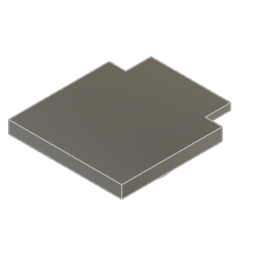
Case (Autodesk Fusion 360 archive; units mm, degrees)
design "Etiquette_game"
Autodesk Fusion 360 part; units mm, degrees
(part 1 of 2)
sketch "Esquisse1" plane through (0, 0, 0) normal (0, 1, 0) x (1, 0, 0)
  line L0 (0, 0) -> (9.5, 0)
  line L1 (9.5, 0) -> (9.5, 0.8)
  line L2 (9.5, 0.8) -> (0, 0.8)
  line L3 (0, 0.8) -> (0, 0)
  dimension "d1" = 9.5
  dimension "d2" = 0.8
  constraint horizontal L0
  constraint vertical L1
  constraint horizontal L2
  constraint vertical L3
  constraint coincident L0.start L3.end
  measures "d1" distance of L0.start L0.end
  measures "d2" distance of L0.start L2.end
extrude "Extrusion1" add sketch "Esquisse1" along normal blind 3
sketch "Esquisse2" plane through (0, 0, 0) normal (0, -1, 0) x (1, 0, 0)
  line L0 (0, 0) -> (0, -0.8)
  line L1 (0, -0.8) -> (9.5, -0.8)
  line L2 (9.5, -0.8) -> (9.5, 0)
  line L3 (9.5, 0) -> (0, 0)
  line L4 (0, 0) -> (-2, 0) construction
  line L5 (9.5, 0) -> (11.5, 0)
  line L6 (11.5, 0) -> (11.5, -1.5)
  line L7 (-2, 0) -> (11.5, 0)
  line L8 (11.5, 0) -> (11.5, -1.5)
  line L9 (11.5, -1.5) -> (-2, -1.5)
  line L10 (-2, -1.5) -> (-2, 0)
  dimension "d5" = 2
  dimension "d6" = 2
  dimension "d7" = 1.5
  constraint coincident L0.start L3.end
  constraint perpendicular L0 L4
  constraint coincident L2.end L3.start
  constraint perpendicular L2 L5
  constraint perpendicular L5 L6
  constraint horizontal L7
  constraint vertical L8
  constraint horizontal L9
  constraint vertical L10
  measures "d5" distance of L0.start L4.end
  measures "d6" distance of L2.end L5.end
  measures "d7" distance of L5.end L6.end
extrude "Extrusion2" add sketch "Esquisse2" along normal blind 12
sketch "Esquisse3" plane through (0, 0, -1.5) normal (0, 0, -1) x (1, 0, 0)
  line L0 (-2, 0) -> (11.5, 0)
  line L1 (11.5, 0) -> (11.5, 12)
  line L2 (11.5, 12) -> (-2, 12)
  line L3 (-2, 12) -> (-2, 0)
  line L4 (0, 6.6162) -> (4, 6.6162)
  line L5 (4, 6.6162) -> (4, 5.4162)
  line L6 (4, 5.4162) -> (0, 5.4162)
  line L7 (0, 5.4162) -> (0, 6.6162)
  line L8 (0, 5.4162) -> (1.4, 5.4162)
  line L9 (1.4, 5.4162) -> (2.6, 5.4162)
  line L10 (2.6, 5.4162) -> (2.6, 4.0162)
  line L11 (2.6, 4.0162) -> (1.4, 4.0162)
  line L12 (1.4, 4.0162) -> (1.4, 5.4162)
  line L13 (1.4, 4.0162) -> (2.6, 4.0162)
  line L14 (2.6, 4.0162) -> (2.6, 8.0162)
  line L15 (2.6, 8.0162) -> (1.4, 8.0162)
  line L16 (1.4, 8.0162) -> (1.4, 4.0162)
  circle A0 centre (6.7088, 5.2403) radius 0.85
  circle A1 centre (8.2624, 6.7784) radius 0.85
  arc A2 (1.5165, 9.1275) -> (4.0468, 3.6361) centre (2.0261, 6.0336) ccw
  line L17 (1.5165, 9.1275) -> (7.8999, 9.1275)
  line L18 (4.0468, 3.6361) -> (5.4235, 3.6361)
  arc A3 (5.4235, 3.6361) -> (7.8999, 9.1275) centre (7.4769, 6.0141) ccw
  dimension "d10" = 4
  dimension "d11" = 1.2
  dimension "d12" = 1.4
  dimension "d13" = 1.2
  dimension "d14" = 1.4
  dimension "d15" = 1.2
  dimension "d16" = 4
  dimension "d17" = 1.7
  dimension "d18" = 1.7
  constraint horizontal L4
  constraint vertical L5
  constraint horizontal L6
  constraint vertical L7
  constraint perpendicular L7 L8
  constraint horizontal L9
  constraint vertical L10
  constraint horizontal L11
  constraint vertical L12
  constraint horizontal L13
  constraint vertical L14
  constraint horizontal L15
  constraint vertical L16
  constraint horizontal L17
  constraint horizontal L18
  measures "d10" distance of L4.start L4.end
  measures "d11" distance of L4.start L6.end
  measures "d12" distance of L6.end L8.end
  measures "d13" distance of L8.end L9.end
  measures "d14" distance of L8.end L11.end
  measures "d15" distance of L11.end L10.end
  measures "d16" distance of L11.end L15.end
  measures "d17" diameter of A0
  measures "d18" diameter of A1
extrude "Extrusion3" add sketch "Esquisse3" along normal blind 1 contours A2 L17 L18 A3

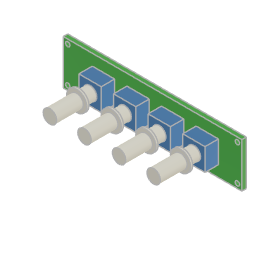
design "PCB_potar"
Autodesk Fusion 360 part; units mm, degrees
sketch "Esquisse1" plane through (0, 0, 0) normal (0, 1, 0) x (1, 0, 0)
  line L0 (0, 0) -> (80, 0)
  line L1 (80, 0) -> (80, 20)
  line L2 (80, 20) -> (0, 20)
  line L3 (0, 20) -> (0, 0)
  line L4 (0, 20) -> (2, 20) construction
  line L5 (2, 20) -> (2, 18) construction
  line L6 (2, 18) -> (0, 18) construction
  line L7 (0, 18) -> (0, 20) construction
  line L8 (0, 0) -> (2, 0) construction
  line L9 (2, 0) -> (2, 2) construction
  line L10 (2, 2) -> (0, 2) construction
  line L11 (0, 2) -> (0, 0) construction
  circle A0 centre (2, 2) radius 1
  circle A1 centre (2, 18) radius 1
  line L12 (40, 20) -> (40, 0) construction
  circle A2 centre (78, 2) radius 1
  circle A3 centre (78, 18) radius 1
  dimension "d1" = 80
  dimension "d2" = 20
  dimension "d20" = 2
  dimension "d21" = 2
  dimension "d22" = 2
  dimension "d23" = 2
  dimension "d24" = 2
  dimension "d25" = 2
  constraint horizontal L0
  constraint vertical L1
  constraint horizontal L2
  constraint vertical L3
  constraint coincident L0.start L3.end
  constraint horizontal L4
  constraint vertical L5
  constraint horizontal L6
  constraint vertical L7
  constraint horizontal L8
  constraint vertical L9
  constraint horizontal L10
  constraint vertical L11
  constraint coincident L9.end L10.start
  constraint coincident L5.end L6.start
  constraint midpoint L2 L12.start
  constraint midpoint L0 L12.end
  constraint symmetric A0 L12 A2
  constraint symmetric A1 L12 A3
  measures "d1" distance of L0.start L0.end
  measures "d2" distance of L0.start L2.end
  measures "d20" distance of L2.end L4.end
  measures "d21" distance of L2.end L6.end
  measures "d22" distance of L0.start L8.end
  measures "d23" distance of L0.start L10.end
  measures "d24" diameter of A0
  measures "d25" diameter of A1
extrude "Extrusion1" add sketch "Esquisse1" along normal blind 2 makes body 1
sketch "Esquisse2" plane through (0, 0, 0) normal (0, -1, 0) x (1, 0, 0)
  line L0 (0, 0) -> (0, -20)
  line L1 (0, -20) -> (80, -20)
  line L2 (80, -20) -> (80, 0)
  line L3 (80, 0) -> (0, 0)
  line L4 (0, 0) -> (13, 0) construction
  line L5 (13, 0) -> (13, -5) construction
  line L6 (13, -5) -> (23, -5)
  line L7 (23, -5) -> (23, -15)
  line L8 (23, -15) -> (13, -15)
  line L9 (13, -15) -> (13, -5)
  line L10 (23, -5) -> (28.5, -5) construction
  line L11 (28.5, -5) -> (38.5, -5)
  line L12 (38.5, -5) -> (38.5, -15)
  line L13 (38.5, -15) -> (28.5, -15)
  line L14 (28.5, -15) -> (28.5, -5)
  line L15 (38.5, -5) -> (44, -5) construction
  line L16 (44, -5) -> (54, -5)
  line L17 (54, -5) -> (54, -15)
  line L18 (54, -15) -> (44, -15)
  line L19 (44, -15) -> (44, -5)
  line L20 (54, -5) -> (59.5, -5) construction
  line L21 (59.5, -5) -> (69.5, -5)
  line L22 (69.5, -5) -> (69.5, -15)
  line L23 (69.5, -15) -> (59.5, -15)
  line L24 (59.5, -15) -> (59.5, -5)
  circle A0 centre (78, -2) radius 1
  circle A1 centre (2, -18) radius 1
  circle A2 centre (2, -2) radius 1
  circle A3 centre (78, -18) radius 1
  dimension "d5" = 13
  dimension "d6" = 5
  dimension "d7" = 10
  dimension "d8" = 10
  dimension "d9" = 5.5
  dimension "d10" = 10
  dimension "d11" = 10
  dimension "d12" = 5.5
  dimension "d13" = 10
  dimension "d14" = 10
  dimension "d15" = 5.5
  dimension "d16" = 10
  dimension "d17" = 10
  constraint coincident L0.start L3.end
  constraint perpendicular L0 L4
  constraint perpendicular L1 L5
  constraint horizontal L6
  constraint vertical L7
  constraint horizontal L8
  constraint vertical L9
  constraint perpendicular L7 L10
  constraint horizontal L11
  constraint vertical L12
  constraint horizontal L13
  constraint vertical L14
  constraint perpendicular L12 L15
  constraint horizontal L16
  constraint vertical L17
  constraint horizontal L18
  constraint vertical L19
  constraint perpendicular L17 L20
  constraint horizontal L21
  constraint vertical L22
  constraint horizontal L23
  constraint vertical L24
  measures "d5" distance of L0.start L4.end
  measures "d6" distance of L4.end L5.end
  measures "d7" distance of L5.end L6.end
  measures "d8" distance of L5.end L8.end
  measures "d9" distance of L6.end L10.end
  measures "d10" distance of L10.end L11.end
  measures "d11" distance of L10.end L13.end
  measures "d12" distance of L11.end L15.end
  measures "d13" distance of L15.end L16.end
  measures "d14" distance of L15.end L18.end
  measures "d15" distance of L16.end L20.end
  measures "d16" distance of L20.end L21.end
  measures "d17" distance of L20.end L23.end
extrude "Extrusion2" add sketch "Esquisse2" along normal blind 6 separate body contours L6 L7 L8 L9 | L11 L12 L13 L14 | L16 L17 L18 L19 | L21 L22 L23 L24 makes body 2 at (31.8333, 0, -8.3333) makes body 3 at (47.3333, 0, -11.6667) makes body 4 at (16.3333, 0, -8.3333) makes body 5 at (62.8333, 0, -8.3333)
sketch "Esquisse3" plane through (0, -6, 0) normal (0, -1, 0) x (1, 0, 0)
  line L0 (13, -15) -> (23, -15)
  line L1 (23, -15) -> (23, -5)
  line L2 (23, -5) -> (13, -5)
  line L3 (13, -5) -> (13, -15)
  line L4 (13, -5) -> (23, -15) construction
  line L5 (13, -15) -> (23, -5) construction
  circle A0 centre (18, -10) radius 3
  dimension "d26" = 6
  constraint coincident L2.end L3.start
  constraint coincident L0.end L1.start
  constraint coincident L0.start L3.end
  constraint coincident L1.end L2.start
  constraint midpoint L5 A0.centre
  measures "d26" diameter of A0
extrude "Extrusion3" add sketch "Esquisse3" along normal blind 5 separate body contours A0 makes body 6
sketch "Esquisse4" plane through (0, -11, 0) normal (0, -1, 0) x (1, 0, 0)
  circle A0 centre (18, -10) radius 3
  circle A1 centre (18, -10) radius 4.5
  dimension "d29" = 9
  constraint concentric A0 A1
  measures "d29" diameter of A1
extrude "Extrusion4" add sketch "Esquisse4" along normal blind 1 contours A0 | A1 bodies 6
sketch "Esquisse5" plane through (0, -12, 0) normal (0, -1, 0) x (1, 0, 0)
  circle A0 centre (18, -10) radius 4.5
  circle A1 centre (18, -10) radius 3
  dimension "d32" = 6
  constraint concentric A0 A1
  measures "d32" diameter of A1
extrude "Extrusion5" add sketch "Esquisse5" along normal blind 12 contours A1 bodies 6
copy_body "Copier/Coller des corps1" bodies 6 makes body 7
move_body "Déplacer1" bodies 7 to x (1, 0, 0) y (0, 1, 0) z (0, 0, 1) at (15.5, 0, 0)
copy_body "Copier/Coller des corps2" bodies 6 makes body 8
move_body "Déplacer2" bodies 8 to x (1, 0, 0) y (0, 1, 0) z (0, 0, 1) at (31, 0, 0)
copy_body "Copier/Coller des corps3" bodies 6 makes body 9
move_body "Déplacer3" bodies 9 to x (1, 0, 0) y (0, 1, 0) z (0, 0, 1) at (46.5, 0, 0)
named bodies: "BASE_PCB", "POTAR_1", "POTAR_2", "POTAR_3", "POTAR_4", "KNOB_1", "KNOB_2", "KNOB_1 (1)", "KNOB_3", "KNOB_1 (2)", "KNOB_4"

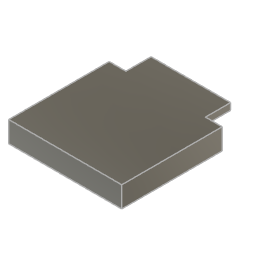
design "Etiquette_deezer"
Autodesk Fusion 360 part; units mm, degrees
sketch "Esquisse1" plane through (0, 0, 0) normal (0, 1, 0) x (1, 0, 0)
  line L0 (0, 0) -> (9.5, 0)
  line L1 (9.5, 0) -> (9.5, 0.8)
  line L2 (9.5, 0.8) -> (0, 0.8)
  line L3 (0, 0.8) -> (0, 0)
  dimension "d1" = 9.5
  dimension "d2" = 0.8
  constraint horizontal L0
  constraint vertical L1
  constraint horizontal L2
  constraint vertical L3
  constraint coincident L0.start L3.end
  measures "d1" distance of L0.start L0.end
  measures "d2" distance of L0.start L2.end
extrude "Extrusion1" add sketch "Esquisse1" along normal blind 3
sketch "Esquisse2" plane through (0, 0, 0) normal (0, -1, 0) x (1, 0, 0)
  line L0 (0, 0) -> (0, -0.8)
  line L1 (0, -0.8) -> (9.5, -0.8)
  line L2 (9.5, -0.8) -> (9.5, 0)
  line L3 (9.5, 0) -> (0, 0)
  line L4 (0, 0) -> (-2, 0) construction
  line L5 (9.5, 0) -> (11.5, 0)
  line L6 (11.5, 0) -> (11.5, -1.5)
  line L7 (-2, 0) -> (11.5, 0)
  line L8 (11.5, 0) -> (11.5, -1.5)
  line L9 (11.5, -1.5) -> (-2, -1.5)
  line L10 (-2, -1.5) -> (-2, 0)
  dimension "d5" = 2
  dimension "d6" = 2
  dimension "d7" = 1.5
  constraint coincident L0.start L3.end
  constraint perpendicular L0 L4
  constraint coincident L2.end L3.start
  constraint perpendicular L2 L5
  constraint perpendicular L5 L6
  constraint horizontal L7
  constraint vertical L8
  constraint horizontal L9
  constraint vertical L10
  measures "d5" distance of L0.start L4.end
  measures "d6" distance of L2.end L5.end
  measures "d7" distance of L5.end L6.end
extrude "Extrusion2" add sketch "Esquisse2" along normal blind 12
sketch "Esquisse3" plane through (0, 0, -1.5) normal (0, 0, -1) x (1, 0, 0)
  line L0 (-2, 0) -> (11.5, 0)
  line L1 (11.5, 0) -> (11.5, 12)
  line L2 (11.5, 12) -> (-2, 12)
  line L3 (-2, 12) -> (-2, 0)
  line L4 (-2, 12) -> (11.5, 0) construction
  line L5 (-2, 0) -> (11.5, 12) construction
  circle A0 centre (4.75, 6) radius 5.5
  line L6 (0.5787, 3.684) -> (2.1287, 3.684)
  line L7 (2.1287, 3.684) -> (2.1287, 4.184)
  line L8 (2.1287, 4.184) -> (0.5787, 4.184)
  line L9 (0.5787, 4.184) -> (0.5787, 3.684)
  line L10 (0.5787, 4.184) -> (0.5787, 4.254)
  line L11 (0.5787, 4.254) -> (2.1287, 4.254)
  line L12 (2.1287, 4.254) -> (2.1287, 4.754)
  line L13 (2.1287, 4.754) -> (0.5787, 4.754)
  line L14 (0.5787, 4.754) -> (0.5787, 4.254)
  line L15 (0.5787, 4.754) -> (0.5787, 4.824)
  line L16 (0.5787, 4.824) -> (2.1287, 4.824)
  line L17 (2.1287, 4.824) -> (2.1287, 5.324)
  line L18 (2.1287, 5.324) -> (0.5787, 5.324)
  line L19 (0.5787, 5.324) -> (0.5787, 4.824)
  line L20 (0.5787, 5.324) -> (0.5787, 5.394)
  line L21 (0.5787, 5.394) -> (2.1287, 5.394)
  line L22 (2.1287, 5.394) -> (2.1287, 5.894)
  line L23 (2.1287, 5.894) -> (0.5787, 5.894)
  line L24 (0.5787, 5.894) -> (0.5787, 5.394)
  line L25 (0.5787, 5.894) -> (0.5787, 5.964)
  line L26 (0.5787, 5.964) -> (2.1287, 5.964)
  line L27 (2.1287, 5.964) -> (2.1287, 6.464)
  line L28 (2.1287, 6.464) -> (0.5787, 6.464)
  line L29 (0.5787, 6.464) -> (0.5787, 5.964)
  line L30 (8.9164, 5.394) -> (8.9164, 5.894)
  line L31 (8.9164, 4.824) -> (8.9164, 5.324)
  line L32 (7.3664, 4.184) -> (7.3664, 3.684)
  line L33 (8.9164, 3.684) -> (8.9164, 4.184)
  line L34 (8.9164, 5.324) -> (7.3664, 5.324)
  line L35 (8.9164, 4.754) -> (7.3664, 4.754)
  line L36 (8.9164, 4.254) -> (8.9164, 4.754)
  line L37 (7.3664, 6.464) -> (7.3664, 5.964)
  line L38 (7.3664, 4.754) -> (7.3664, 4.254)
  line L39 (7.3664, 5.894) -> (7.3664, 5.394)
  line L40 (8.9164, 5.964) -> (8.9164, 6.464)
  line L41 (7.3664, 4.754) -> (7.3664, 4.824)
  line L42 (7.3664, 5.324) -> (7.3664, 5.394)
  line L43 (7.3664, 5.324) -> (7.3664, 4.824)
  line L44 (8.9164, 5.894) -> (7.3664, 5.894)
  line L45 (7.3664, 3.684) -> (8.9164, 3.684)
  line L46 (7.3664, 4.254) -> (8.9164, 4.254)
  line L47 (7.3664, 5.394) -> (8.9164, 5.394)
  line L48 (7.3664, 4.824) -> (8.9164, 4.824)
  line L49 (7.3664, 4.184) -> (7.3664, 4.254)
  line L50 (8.9164, 4.184) -> (7.3664, 4.184)
  line L51 (8.9164, 6.464) -> (7.3664, 6.464)
  line L52 (7.3664, 5.894) -> (7.3664, 5.964)
  line L53 (7.3664, 5.964) -> (8.9164, 5.964)
  line L54 (5.5066, 5.394) -> (5.5066, 5.894)
  line L55 (5.5066, 4.824) -> (5.5066, 5.324)
  line L56 (3.9566, 4.184) -> (3.9566, 3.684)
  line L57 (5.5066, 3.684) -> (5.5066, 4.184)
  line L58 (5.5066, 5.324) -> (3.9566, 5.324)
  line L59 (5.5066, 4.754) -> (3.9566, 4.754)
  line L60 (5.5066, 4.254) -> (5.5066, 4.754)
  line L61 (3.9566, 6.464) -> (3.9566, 5.964)
  line L62 (3.9566, 4.754) -> (3.9566, 4.254)
  line L63 (3.9566, 5.894) -> (3.9566, 5.394)
  line L64 (5.5066, 5.964) -> (5.5066, 6.464)
  line L65 (3.9566, 4.754) -> (3.9566, 4.824)
  line L66 (3.9566, 5.324) -> (3.9566, 5.394)
  line L67 (3.9566, 5.324) -> (3.9566, 4.824)
  line L68 (5.5066, 5.894) -> (3.9566, 5.894)
  line L69 (3.9566, 3.684) -> (5.5066, 3.684)
  line L70 (3.9566, 4.254) -> (5.5066, 4.254)
  line L71 (3.9566, 5.394) -> (5.5066, 5.394)
  line L72 (3.9566, 4.824) -> (5.5066, 4.824)
  line L73 (3.9566, 4.184) -> (3.9566, 4.254)
  line L74 (5.5066, 4.184) -> (3.9566, 4.184)
  line L75 (5.5066, 6.464) -> (3.9566, 6.464)
  line L76 (3.9566, 5.894) -> (3.9566, 5.964)
  line L77 (3.9566, 5.964) -> (5.5066, 5.964)
  line L78 (7.1756, 5.394) -> (7.1756, 5.894)
  line L79 (7.1756, 4.824) -> (7.1756, 5.324)
  line L80 (5.6256, 4.184) -> (5.6256, 3.684)
  line L81 (7.1756, 3.684) -> (7.1756, 4.184)
  line L82 (7.1756, 5.324) -> (5.6256, 5.324)
  line L83 (7.1756, 4.754) -> (5.6256, 4.754)
  line L84 (7.1756, 4.254) -> (7.1756, 4.754)
  line L85 (5.6256, 6.464) -> (5.6256, 5.964)
  line L86 (5.6256, 4.754) -> (5.6256, 4.254)
  line L87 (5.6256, 5.894) -> (5.6256, 5.394)
  line L88 (7.1756, 5.964) -> (7.1756, 6.464)
  line L89 (5.6256, 4.754) -> (5.6256, 4.824)
  line L90 (5.6256, 5.324) -> (5.6256, 5.394)
  line L91 (5.6256, 5.324) -> (5.6256, 4.824)
  line L92 (7.1756, 5.894) -> (5.6256, 5.894)
  line L93 (5.6256, 3.684) -> (7.1756, 3.684)
  line L94 (5.6256, 4.254) -> (7.1756, 4.254)
  line L95 (5.6256, 5.394) -> (7.1756, 5.394)
  line L96 (5.6256, 4.824) -> (7.1756, 4.824)
  line L97 (5.6256, 4.184) -> (5.6256, 4.254)
  line L98 (7.1756, 4.184) -> (5.6256, 4.184)
  line L99 (7.1756, 6.464) -> (5.6256, 6.464)
  line L100 (5.6256, 5.894) -> (5.6256, 5.964)
  line L101 (5.6256, 5.964) -> (7.1756, 5.964)
  line L102 (3.8376, 5.394) -> (3.8376, 5.894)
  line L103 (3.8376, 4.824) -> (3.8376, 5.324)
  line L104 (2.2876, 4.184) -> (2.2876, 3.684)
  line L105 (3.8376, 3.684) -> (3.8376, 4.184)
  line L106 (3.8376, 5.324) -> (2.2876, 5.324)
  line L107 (3.8376, 4.754) -> (2.2876, 4.754)
  line L108 (3.8376, 4.254) -> (3.8376, 4.754)
  line L109 (2.2876, 6.464) -> (2.2876, 5.964)
  line L110 (2.2876, 4.754) -> (2.2876, 4.254)
  line L111 (2.2876, 5.894) -> (2.2876, 5.394)
  line L112 (3.8376, 5.964) -> (3.8376, 6.464)
  line L113 (2.2876, 4.754) -> (2.2876, 4.824)
  line L114 (2.2876, 5.324) -> (2.2876, 5.394)
  line L115 (2.2876, 5.324) -> (2.2876, 4.824)
  line L116 (3.8376, 5.894) -> (2.2876, 5.894)
  line L117 (2.2876, 3.684) -> (3.8376, 3.684)
  line L118 (2.2876, 4.254) -> (3.8376, 4.254)
  line L119 (2.2876, 5.394) -> (3.8376, 5.394)
  line L120 (2.2876, 4.824) -> (3.8376, 4.824)
  line L121 (2.2876, 4.184) -> (2.2876, 4.254)
  line L122 (3.8376, 4.184) -> (2.2876, 4.184)
  line L123 (3.8376, 6.464) -> (2.2876, 6.464)
  line L124 (2.2876, 5.894) -> (2.2876, 5.964)
  line L125 (2.2876, 5.964) -> (3.8376, 5.964)
  line L126 (5.507, 5.3964) -> (5.507, 5.8964)
  line L127 (3.957, 4.8264) -> (5.507, 4.8264)
  line L128 (5.507, 5.3264) -> (3.957, 5.3264)
  line L129 (5.507, 4.8264) -> (5.507, 5.3264)
  line L130 (3.957, 7.1064) -> (5.507, 7.1064)
  line L131 (3.957, 6.4664) -> (3.957, 6.5364)
  line L132 (5.507, 7.6064) -> (3.957, 7.6064)
  line L133 (5.507, 6.5364) -> (5.507, 7.0364)
  line L134 (3.957, 7.6064) -> (3.957, 7.1064)
  line L135 (5.507, 6.4664) -> (3.957, 6.4664)
  line L136 (5.507, 7.0364) -> (3.957, 7.0364)
  line L137 (5.507, 5.8964) -> (3.957, 5.8964)
  line L138 (3.957, 5.3964) -> (5.507, 5.3964)
  line L139 (5.507, 7.1064) -> (5.507, 7.6064)
  line L140 (3.957, 7.0364) -> (3.957, 6.5364)
  line L141 (3.957, 7.0364) -> (3.957, 7.1064)
  line L142 (3.957, 6.4664) -> (3.957, 5.9664)
  line L143 (3.957, 5.9664) -> (5.507, 5.9664)
  line L144 (3.957, 5.8964) -> (3.957, 5.9664)
  line L145 (3.957, 5.3264) -> (3.957, 5.3964)
  line L146 (5.507, 5.9664) -> (5.507, 6.4664)
  line L147 (3.957, 5.8964) -> (3.957, 5.3964)
  line L148 (3.957, 5.3264) -> (3.957, 4.8264)
  line L149 (3.957, 6.5364) -> (5.507, 6.5364)
  line L150 (8.9062, 7.2438) -> (8.9062, 7.7438)
  line L151 (7.3562, 6.6738) -> (8.9062, 6.6738)
  line L152 (8.9062, 7.1738) -> (7.3562, 7.1738)
  line L153 (8.9062, 6.6738) -> (8.9062, 7.1738)
  line L154 (7.3562, 8.9538) -> (8.9062, 8.9538)
  line L155 (7.3562, 8.3138) -> (7.3562, 8.3838)
  line L156 (8.9062, 9.4538) -> (7.3562, 9.4538)
  line L157 (8.9062, 8.3838) -> (8.9062, 8.8838)
  line L158 (7.3562, 9.4538) -> (7.3562, 8.9538)
  line L159 (8.9062, 8.3138) -> (7.3562, 8.3138)
  line L160 (8.9062, 8.8838) -> (7.3562, 8.8838)
  line L161 (8.9062, 7.7438) -> (7.3562, 7.7438)
  line L162 (7.3562, 7.2438) -> (8.9062, 7.2438)
  line L163 (8.9062, 8.9538) -> (8.9062, 9.4538)
  line L164 (7.3562, 8.8838) -> (7.3562, 8.3838)
  line L165 (7.3562, 8.8838) -> (7.3562, 8.9538)
  line L166 (7.3562, 8.3138) -> (7.3562, 7.8138)
  line L167 (7.3562, 7.8138) -> (8.9062, 7.8138)
  line L168 (7.3562, 7.7438) -> (7.3562, 7.8138)
  line L169 (7.3562, 7.1738) -> (7.3562, 7.2438)
  line L170 (8.9062, 7.8138) -> (8.9062, 8.3138)
  line L171 (7.3562, 7.7438) -> (7.3562, 7.2438)
  line L172 (7.3562, 7.1738) -> (7.3562, 6.6738)
  line L173 (7.3562, 8.3838) -> (8.9062, 8.3838)
  dimension "d10" = 11
  dimension "d11" = 1.55
  dimension "d12" = 0.5
  dimension "d13" = 0.07
  dimension "d14" = 1.55
  dimension "d15" = 0.5
  dimension "d16" = 0.07
  dimension "d17" = 1.55
  dimension "d18" = 0.5
  dimension "d19" = 0.07
  dimension "d20" = 1.55
  dimension "d21" = 0.5
  dimension "d22" = 0.07
  dimension "d23" = 1.55
  dimension "d24" = 0.5
  dimension "d25" = 0.07
  dimension "d26" = 1.55
  dimension "d27" = 0.5
  dimension "d28" = 0.07
  dimension "d29" = 1.55
  dimension "d30" = 0.5
  dimension "d31" = 0.07
  constraint coincident L2.end L3.start
  constraint coincident L0.end L1.start
  constraint coincident L0.start L3.end
  constraint coincident L1.end L2.start
  constraint midpoint L4 A0.centre
  constraint horizontal L6
  constraint vertical L7
  constraint horizontal L8
  constraint vertical L9
  constraint perpendicular L8 L10
  constraint horizontal L11
  constraint vertical L12
  constraint horizontal L13
  constraint vertical L14
  constraint perpendicular L13 L15
  constraint horizontal L16
  constraint vertical L17
  constraint horizontal L18
  constraint vertical L19
  constraint perpendicular L18 L20
  constraint horizontal L21
  constraint vertical L22
  constraint horizontal L23
  constraint vertical L24
  constraint perpendicular L23 L25
  constraint horizontal L26
  constraint vertical L27
  constraint horizontal L28
  constraint vertical L29
  constraint equal L10 L15
  constraint equal L20 L25
  constraint equal L15 L20
  constraint equal L7 L12
  constraint equal L12 L17
  constraint equal L17 L22
  constraint equal L22 L27
  constraint equal L23 L28
  constraint equal L13 L18
  constraint equal L8 L11
  constraint equal L18 L21
  constraint horizontal L45
  constraint vertical L33
  constraint horizontal L50
  constraint vertical L32
  constraint perpendicular L49 L50
  constraint horizontal L46
  constraint vertical L36
  constraint horizontal L35
  constraint vertical L38
  constraint perpendicular L35 L41
  constraint horizontal L48
  constraint vertical L31
  constraint horizontal L34
  constraint vertical L43
  constraint perpendicular L34 L42
  constraint horizontal L47
  constraint vertical L30
  constraint horizontal L44
  constraint vertical L39
  constraint perpendicular L44 L52
  constraint horizontal L53
  constraint vertical L40
  constraint horizontal L51
  constraint vertical L37
  constraint equal L41 L49
  constraint equal L42 L52
  constraint equal L41 L42
  constraint equal L33 L36
  constraint equal L31 L36
  constraint equal L30 L31
  constraint equal L30 L40
  constraint equal L44 L51
  constraint equal L34 L35
  constraint equal L46 L50
  constraint equal L34 L47
  constraint horizontal L69
  constraint vertical L57
  constraint horizontal L74
  constraint vertical L56
  constraint perpendicular L73 L74
  constraint horizontal L70
  constraint vertical L60
  constraint horizontal L59
  constraint vertical L62
  constraint perpendicular L59 L65
  constraint horizontal L72
  constraint vertical L55
  constraint horizontal L58
  constraint vertical L67
  constraint perpendicular L58 L66
  constraint horizontal L71
  constraint vertical L54
  constraint horizontal L68
  constraint vertical L63
  constraint perpendicular L68 L76
  constraint horizontal L77
  constraint vertical L64
  constraint horizontal L75
  constraint vertical L61
  constraint equal L65 L73
  constraint equal L66 L76
  constraint equal L65 L66
  constraint equal L57 L60
  constraint equal L55 L60
  constraint equal L54 L55
  constraint equal L54 L64
  constraint equal L68 L75
  constraint equal L58 L59
  constraint equal L70 L74
  constraint equal L58 L71
  constraint horizontal L93
  constraint vertical L81
  constraint horizontal L98
  constraint vertical L80
  constraint perpendicular L97 L98
  constraint horizontal L94
  constraint vertical L84
  constraint horizontal L83
  constraint vertical L86
  constraint perpendicular L83 L89
  constraint horizontal L96
  constraint vertical L79
  constraint horizontal L82
  constraint vertical L91
  constraint perpendicular L82 L90
  constraint horizontal L95
  constraint vertical L78
  constraint horizontal L92
  constraint vertical L87
  constraint perpendicular L92 L100
  constraint horizontal L101
  constraint vertical L88
  constraint horizontal L99
  constraint vertical L85
  constraint equal L89 L97
  constraint equal L90 L100
  constraint equal L89 L90
  constraint equal L81 L84
  constraint equal L79 L84
  constraint equal L78 L79
  constraint equal L78 L88
  constraint equal L92 L99
  constraint equal L82 L83
  constraint equal L94 L98
  constraint equal L82 L95
  constraint horizontal L117
  constraint vertical L105
  constraint horizontal L122
  constraint vertical L104
  constraint perpendicular L121 L122
  constraint horizontal L118
  constraint vertical L108
  constraint horizontal L107
  constraint vertical L110
  constraint perpendicular L107 L113
  constraint horizontal L120
  constraint vertical L103
  constraint horizontal L106
  constraint vertical L115
  constraint perpendicular L106 L114
  constraint horizontal L119
  constraint vertical L102
  constraint horizontal L116
  constraint vertical L111
  constraint perpendicular L116 L124
  constraint horizontal L125
  constraint vertical L112
  constraint horizontal L123
  constraint vertical L109
  constraint equal L113 L121
  constraint equal L114 L124
  constraint equal L113 L114
  constraint equal L105 L108
  constraint equal L103 L108
  constraint equal L102 L103
  constraint equal L102 L112
  constraint equal L116 L123
  constraint equal L106 L107
  constraint equal L118 L122
  constraint equal L106 L119
  constraint horizontal L127
  constraint vertical L129
  constraint horizontal L128
  constraint vertical L148
  constraint perpendicular L128 L145
  constraint horizontal L138
  constraint vertical L126
  constraint horizontal L137
  constraint vertical L147
  constraint perpendicular L137 L144
  constraint horizontal L143
  constraint vertical L146
  constraint horizontal L135
  constraint vertical L142
  constraint perpendicular L131 L135
  constraint horizontal L149
  constraint vertical L133
  constraint horizontal L136
  constraint vertical L140
  constraint perpendicular L136 L141
  constraint horizontal L130
  constraint vertical L139
  constraint horizontal L132
  constraint vertical L134
  constraint equal L144 L145
  constraint equal L131 L141
  constraint equal L131 L144
  constraint equal L126 L129
  constraint equal L126 L146
  constraint equal L133 L146
  constraint equal L133 L139
  constraint equal L132 L136
  constraint equal L135 L137
  constraint equal L128 L138
  constraint equal L135 L149
  constraint horizontal L151
  constraint vertical L153
  constraint horizontal L152
  constraint vertical L172
  constraint perpendicular L152 L169
  constraint horizontal L162
  constraint vertical L150
  constraint horizontal L161
  constraint vertical L171
  constraint perpendicular L161 L168
  constraint horizontal L167
  constraint vertical L170
  constraint horizontal L159
  constraint vertical L166
  constraint perpendicular L155 L159
  constraint horizontal L173
  constraint vertical L157
  constraint horizontal L160
  constraint vertical L164
  constraint perpendicular L160 L165
  constraint horizontal L154
  constraint vertical L163
  constraint horizontal L156
  constraint vertical L158
  constraint equal L168 L169
  constraint equal L155 L165
  constraint equal L155 L168
  constraint equal L150 L153
  constraint equal L150 L170
  constraint equal L157 L170
  constraint equal L157 L163
  constraint equal L156 L160
  constraint equal L159 L161
  constraint equal L152 L162
  constraint equal L159 L173
  measures "d10" diameter of A0
  measures "d11" distance of L6.start L6.end
  measures "d12" distance of L6.start L8.end
  measures "d13" distance of L8.end L10.end
  measures "d14" distance of L32.end L33.start
  measures "d15" distance of L32.end L32.start
  measures "d16" distance of L32.start L38.end
  measures "d17" distance of L56.end L57.start
  measures "d18" distance of L56.end L56.start
  measures "d19" distance of L56.start L62.end
  measures "d20" distance of L80.end L81.start
  measures "d21" distance of L80.end L80.start
  measures "d22" distance of L80.start L86.end
  measures "d23" distance of L104.end L105.start
  measures "d24" distance of L104.end L104.start
  measures "d25" distance of L104.start L110.end
  measures "d26" distance of L127.start L127.end
  measures "d27" distance of L127.start L128.end
  measures "d28" distance of L128.end L138.start
  measures "d29" distance of L151.start L151.end
  measures "d30" distance of L151.start L152.end
  measures "d31" distance of L152.end L162.start
extrude "Extrusion3" add sketch "Esquisse3" along normal blind 1 contours L0 L1 L2 L3 | L6 L7 L8 L9 | L11 L12 L13 L14 | L16 L17 L18 L19 | L21 L22 L23 L24 | L26 L27 L28 L29 | L30 L39 L44 L47 | L31 L34 L43 L48 | L32 L33 L45 L50 | L35 L36 L38 L46 | L37 L40 L51 L53 | L54 L68 L138 L147 | L55 L58 L127 L148 | L64 L75 L142 L143 | L56 L57 L69 L74 | L59 L60 L62 L70 | L78 L87 L92 L95 | L79 L82 L91 L96 | L80 L81 L93 L98 | L83 L84 L86 L94 | L85 L88 L99 L101 | L103 L106 L115 L120 | L104 L105 L117 L122 | L107 L108 L110 L118 | L130 L132 L134 L139 | L133 L136 L140 L149 | L150 L161 L162 L171 | L151 L152 L153 L172 | L159 L166 L167 L170

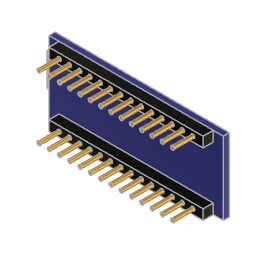
design "Arduino_nano"
Autodesk Fusion 360 part; units mm, degrees
sketch "Esquisse1" plane through (0, 0, 0) normal (0, 1, 0) x (1, 0, 0)
  line L0 (0, 0) -> (43, 0)
  line L1 (43, 0) -> (43, 18)
  line L2 (43, 18) -> (0, 18)
  line L3 (0, 18) -> (0, 0)
  dimension "d1" = 43
  dimension "d2" = 18
  constraint horizontal L0
  constraint vertical L1
  constraint horizontal L2
  constraint vertical L3
  constraint coincident L0.start L3.end
  measures "d1" distance of L0.start L0.end
  measures "d2" distance of L0.start L2.end
extrude "Extrusion1" add sketch "Esquisse1" along normal blind 1.5 makes body 1
sketch "Esquisse2" plane through (0, 0, 0) normal (0, -1, 0) x (1, 0, 0)
  line L0 (0, 0) -> (0, -18)
  line L1 (0, -18) -> (43, -18)
  line L2 (43, -18) -> (43, 0)
  line L3 (43, 0) -> (0, 0)
  line L4 (0, 0) -> (43, 0)
  line L5 (43, 0) -> (43, -2.5)
  line L6 (43, -2.5) -> (0, -2.5)
  line L7 (0, -2.5) -> (0, 0)
  line L8 (0, -18) -> (43, -18)
  line L9 (43, -18) -> (43, -15.5)
  line L10 (43, -15.5) -> (0, -15.5)
  line L11 (0, -15.5) -> (0, -18)
  line L12 (0, 0) -> (2.5, 0)
  line L13 (2.5, 0) -> (2.5, -18)
  line L14 (2.5, -18) -> (0, -18)
  line L15 (0, -18) -> (0, 0)
  line L16 (43, -18) -> (40.5, -18)
  line L17 (40.5, -18) -> (40.5, 0)
  line L18 (40.5, 0) -> (43, 0)
  line L19 (43, 0) -> (43, -18)
  dimension "d5" = 2.5
  dimension "d6" = 2.5
  dimension "d9" = 2.5
  dimension "d10" = 2.5
  constraint horizontal L4
  constraint vertical L5
  constraint horizontal L6
  constraint vertical L7
  constraint coincident L0.start L3.end
  constraint horizontal L8
  constraint vertical L9
  constraint horizontal L10
  constraint vertical L11
  constraint coincident L0.end L1.start
  constraint horizontal L12
  constraint vertical L13
  constraint horizontal L14
  constraint vertical L15
  constraint coincident L8 L13.end
  constraint horizontal L16
  constraint vertical L17
  constraint horizontal L18
  constraint vertical L19
  measures "d5" distance of L0.start L6.end
  measures "d6" distance of L0.end L10.end
  measures "d9" distance of L0.start L12.end
  measures "d10" distance of L1.end L16.end
extrude "Extrusion2" add sketch "Esquisse2" along normal blind 2.5 separate body contours L3 L4 L6 L13 L17 | L1 L8 L10 L13 L17 makes body 2 at (27.8333, -0.8333, 0) makes body 3 at (27.8333, -0.8333, -15.5)
sketch "Esquisse3" plane through (0, -2.5, 0) normal (0, -1, 0) x (1, 0, 0)
  line L0 (2.5, 0) -> (2.5, -2.5)
  line L1 (2.5, -2.5) -> (40.5, -2.5)
  line L2 (40.5, -2.5) -> (40.5, 0)
  line L3 (40.5, 0) -> (2.5, 0)
  line L4 (40.5, -1.25) -> (37.9667, -1.25) construction
  circle A0 centre (37.9667, -1.25) radius 0.5
  line L5 (37.9667, -1.25) -> (35.4333, -1.25) construction
  line L6 (35.4333, -1.25) -> (32.9, -1.25) construction
  line L7 (32.9, -1.25) -> (30.3667, -1.25) construction
  line L8 (30.3667, -1.25) -> (27.8333, -1.25) construction
  line L9 (27.8333, -1.25) -> (25.3, -1.25) construction
  line L10 (25.3, -1.25) -> (22.7667, -1.25) construction
  line L11 (22.7667, -1.25) -> (20.2333, -1.25) construction
  line L12 (20.2333, -1.25) -> (17.7, -1.25) construction
  line L13 (17.7, -1.25) -> (15.1667, -1.25) construction
  line L14 (15.1667, -1.25) -> (12.6333, -1.25) construction
  line L15 (12.6333, -1.25) -> (10.1, -1.25) construction
  line L16 (10.1, -1.25) -> (7.5667, -1.25) construction
  line L17 (7.5667, -1.25) -> (5.0333, -1.25) construction
  line L18 (5.0333, -1.25) -> (2.5, -1.25) construction
  circle A1 centre (5.0333, -1.25) radius 0.5
  circle A2 centre (7.5667, -1.25) radius 0.5
  circle A3 centre (10.1, -1.25) radius 0.5
  circle A4 centre (12.6333, -1.25) radius 0.5
  circle A5 centre (15.1667, -1.25) radius 0.5
  circle A6 centre (17.7, -1.25) radius 0.5
  circle A7 centre (20.2333, -1.25) radius 0.5
  circle A8 centre (22.7667, -1.25) radius 0.5
  circle A9 centre (25.3, -1.25) radius 0.5
  circle A10 centre (27.8333, -1.25) radius 0.5
  circle A11 centre (30.3667, -1.25) radius 0.5
  circle A12 centre (32.9, -1.25) radius 0.5
  circle A13 centre (35.4333, -1.25) radius 0.5
  line L19 (0, 0) -> (43, 0)
  line L20 (43, 0) -> (43, -18)
  line L21 (43, -18) -> (0, -18)
  line L22 (0, -18) -> (0, 0)
  line L23 (0, -9) -> (43, -9) construction
  circle A14 centre (5.0333, -16.75) radius 0.5
  circle A15 centre (7.5667, -16.75) radius 0.5
  circle A16 centre (10.1, -16.75) radius 0.5
  circle A17 centre (12.6333, -16.75) radius 0.5
  circle A18 centre (15.1667, -16.75) radius 0.5
  circle A19 centre (17.7, -16.75) radius 0.5
  circle A20 centre (20.2333, -16.75) radius 0.5
  circle A21 centre (22.7667, -16.75) radius 0.5
  circle A22 centre (25.3, -16.75) radius 0.5
  circle A23 centre (27.8333, -16.75) radius 0.5
  circle A24 centre (30.3667, -16.75) radius 0.5
  circle A25 centre (32.9, -16.75) radius 0.5
  circle A26 centre (35.4333, -16.75) radius 0.5
  circle A27 centre (37.9667, -16.75) radius 0.5
  dimension "d11" = 2.5333
  dimension "d12" = 1
  dimension "d13" = 2.5333
  dimension "d14" = 2.5333
  dimension "d15" = 2.5333
  dimension "d16" = 2.5333
  dimension "d17" = 2.5333
  dimension "d18" = 2.5333
  dimension "d19" = 2.5333
  dimension "d20" = 2.5333
  dimension "d21" = 2.5333
  dimension "d22" = 2.5333
  dimension "d23" = 2.5333
  dimension "d24" = 2.5333
  dimension "d25" = 2.5333
  dimension "d26" = 2.5333
  dimension "d27" = 43
  dimension "d28" = 18
  constraint midpoint L2 L4.start
  constraint perpendicular L2 L4
  constraint coincident L4.end A0.centre
  constraint parallel L4 L5
  constraint parallel L5 L6
  constraint parallel L6 L7
  constraint parallel L7 L8
  constraint parallel L8 L9
  constraint parallel L9 L10
  constraint parallel L10 L11
  constraint parallel L11 L12
  constraint parallel L11 L13
  constraint parallel L11 L14
  constraint parallel L11 L15
  constraint parallel L11 L16
  constraint parallel L11 L17
  constraint parallel L11 L18
  constraint coincident L17.end L18.start
  constraint coincident L16.end L17.start
  constraint coincident L15.end L16.start
  constraint coincident L14.end L15.start
  constraint coincident L13.end L14.start
  constraint coincident L12.end L13.start
  constraint coincident L11.end L12.start
  constraint coincident L10.end L11.start
  constraint coincident L9.end L10.start
  constraint coincident L8.end L9.start
  constraint coincident L7.end L8.start
  constraint coincident L6.end L7.start
  constraint coincident L5.end L6.start
  constraint equal A0 A13
  constraint equal A12 A13
  constraint equal A11 A12
  constraint equal A10 A11
  constraint equal A9 A10
  constraint equal A8 A9
  constraint equal A7 A8
  constraint equal A6 A7
  constraint equal A5 A6
  constraint equal A4 A5
  constraint equal A3 A4
  constraint equal A2 A3
  constraint equal A1 A2
  constraint horizontal L19
  constraint vertical L20
  constraint horizontal L21
  constraint vertical L22
  constraint coincident L19.start L22.end
  constraint midpoint L22 L23.start
  constraint midpoint L20 L23.end
  constraint symmetric A0 L23 A27
  constraint symmetric A1 L23 A14
  constraint symmetric A2 L23 A15
  constraint symmetric A3 L23 A16
  constraint symmetric A4 L23 A17
  constraint symmetric A5 L23 A18
  constraint symmetric A6 L23 A19
  constraint symmetric A7 L23 A20
  constraint symmetric A8 L23 A21
  constraint symmetric A9 L23 A22
  constraint symmetric A10 L23 A23
  constraint symmetric A11 L23 A24
  constraint symmetric A12 L23 A25
  constraint symmetric A13 L23 A26
  measures "d11" distance of L4.start L4.end
  measures "d12" diameter of A0
  measures "d13" distance of L4.end L5.end
  measures "d14" distance of L5.end L6.end
  measures "d15" distance of L6.end L7.end
  measures "d16" distance of L7.end L8.end
  measures "d17" distance of L8.end L9.end
  measures "d18" distance of L9.end L10.end
  measures "d19" distance of L10.end L11.end
  measures "d20" distance of L11.end L12.end
  measures "d21" distance of L12.end L13.end
  measures "d22" distance of L13.end L14.end
  measures "d23" distance of L14.end L15.end
  measures "d24" distance of L15.end L16.end
  measures "d25" distance of L16.end L17.end
  measures "d26" distance of L17.end L18.end
  measures "d27" distance of L19.start L19.end
  measures "d28" distance of L19.start L21.end
extrude "Extrusion1'" add sketch "Esquisse3" along normal blind 5 separate body contours A0 | A1 | A2 | A3 | A4 | A5 | A6 | A7 | A8 | A9 | A10 | A11 | A12 | A13 | A14 | A15 | A16 | A17 | A18 | A19 | A20 | A21 | A22 | A23 | A24 | A25 | A26 | A27 makes body 4 at (33.3698, -5.8333, -16.579) makes body 5 at (23.2365, -5.8333, -16.579) makes body 6 at (13.1032, -5.8333, -16.579) makes body 7 at (38.2379, -5.8333, -0.83) makes body 8 at (28.1046, -5.8333, -0.83) makes body 9 at (17.9713, -5.8333, -0.83) makes body 10 at (8.066, -5.8333, -1.2749) makes body 11 at (10.5994, -5.8333, -1.2749) makes body 12 at (20.5046, -5.8333, -0.83) makes body 13 at (30.6379, -5.8333, -0.83) makes body 14 at (5.5032, -5.8333, -16.579) makes body 15 at (15.6365, -5.8333, -16.579) makes body 16 at (25.7698, -5.8333, -16.579) makes body 17 at (35.9032, -5.8333, -16.579) makes body 18 at (30.8365, -5.8333, -16.579) makes body 19 at (20.7032, -5.8333, -16.579) makes body 20 at (10.5698, -5.8333, -16.579) makes body 21 at (35.7046, -5.8333, -0.83) makes body 22 at (25.5713, -5.8333, -0.83) makes body 23 at (15.666, -5.8333, -1.2749) makes body 24 at (5.5327, -5.8333, -1.2749) makes body 25 at (13.1327, -5.8333, -1.2749) makes body 26 at (23.0379, -5.8333, -0.83) makes body 27 at (33.1713, -5.8333, -0.83) makes body 28 at (8.0365, -5.8333, -16.579) makes body 29 at (18.1698, -5.8333, -16.579) makes body 30 at (28.3032, -5.8333, -16.579) makes body 31 at (38.4365, -5.8333, -16.579) in component "Component"
sketch "Esquisse4" plane through (0, 1.5, 0) normal (0, 1, 0) x (-1, 0, 0)
  line L0 (0, -18) -> (0, 0)
  line L1 (0, 0) -> (-43, 0)
  line L2 (-43, 0) -> (-43, -18)
  line L3 (-43, -18) -> (0, -18)
  line L4 (0, 0) -> (2, 0)
  line L5 (2, 0) -> (2, -5)
  line L6 (2, -5) -> (0.0623, -5)
  line L7 (0.0623, -5) -> (0.0623, -13)
  line L8 (0.0623, -13) -> (2, -13)
  line L9 (2, -13) -> (2, -5)
  line L10 (2, -13) -> (-7, -13)
  line L11 (-7, -13) -> (-7, -5)
  line L12 (-7, -5) -> (2, -5)
  line L13 (2, -5) -> (2, -13)
  dimension "d31" = 2
  dimension "d32" = 5
  dimension "d33" = 8
  dimension "d34" = 9
  dimension "d35" = 8
  constraint coincident L0.end L1.start
  constraint perpendicular L0 L4
  constraint perpendicular L1 L5
  constraint horizontal L6
  constraint vertical L7
  constraint horizontal L8
  constraint vertical L9
  constraint horizontal L10
  constraint vertical L11
  constraint horizontal L12
  constraint vertical L13
  measures "d31" distance of L0.end L4.end
  measures "d32" distance of L4.end L5.end
  measures "d33" distance of L5.end L8.end
  measures "d34" distance of L8.end L10.end
  measures "d35" distance of L8.end L5.end
extrude "Extrusion3" add sketch "Esquisse4" along normal blind 4 separate body contours L0 L10 L11 L12 | L0 L7 L10 L12 | L6 L7 L8 L9 L10 L12 L13 makes body 32
component "Component" placed x (1, 0, 0) y (0, 1, 0) z (0, 0, 1) at (0, 0, 0)
equation "d11 = ( 38 / 15 ) * 1 mm"
equation "d13 = ( 38 / 15 ) * 1 mm"
equation "d14 = ( 38 / 15 ) * 1 mm"
equation "d15 = ( 38 / 15 ) * 1 mm"
equation "d16 = ( 38 / 15 ) * 1 mm"
equation "d17 = ( 38 / 15 ) * 1 mm"
equation "d18 = ( 38 / 15 ) * 1 mm"
equation "d19 = ( 38 / 15 ) * 1 mm"
equation "d20 = ( 38 / 15 ) * 1 mm"
equation "d21 = ( 38 / 15 ) * 1 mm"
equation "d22 = ( 38 / 15 ) * 1 mm"
equation "d23 = ( 38 / 15 ) * 1 mm"
equation "d24 = ( 38 / 15 ) * 1 mm"
equation "d26 = ( 38 / 15 ) * 1 mm"

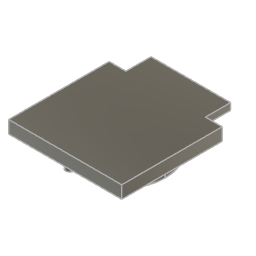
design "Etiquette_general"
Autodesk Fusion 360 part; units mm, degrees
sketch "Esquisse1" plane through (0, 0, 0) normal (0, 1, 0) x (1, 0, 0)
  line L0 (0, 0) -> (9.5, 0)
  line L1 (9.5, 0) -> (9.5, 0.8)
  line L2 (9.5, 0.8) -> (0, 0.8)
  line L3 (0, 0.8) -> (0, 0)
  dimension "d1" = 9.5
  dimension "d2" = 0.8
  constraint horizontal L0
  constraint vertical L1
  constraint horizontal L2
  constraint vertical L3
  constraint coincident L0.start L3.end
  measures "d1" distance of L0.start L0.end
  measures "d2" distance of L0.start L2.end
extrude "Extrusion1" add sketch "Esquisse1" along normal blind 3
sketch "Esquisse2" plane through (0, 0, 0) normal (0, -1, 0) x (1, 0, 0)
  line L0 (0, 0) -> (0, -0.8)
  line L1 (0, -0.8) -> (9.5, -0.8)
  line L2 (9.5, -0.8) -> (9.5, 0)
  line L3 (9.5, 0) -> (0, 0)
  line L4 (0, 0) -> (-2, 0) construction
  line L5 (9.5, 0) -> (11.5, 0)
  line L6 (11.5, 0) -> (11.5, -1.5)
  line L7 (-2, 0) -> (11.5, 0)
  line L8 (11.5, 0) -> (11.5, -1.5)
  line L9 (11.5, -1.5) -> (-2, -1.5)
  line L10 (-2, -1.5) -> (-2, 0)
  dimension "d5" = 2
  dimension "d6" = 2
  dimension "d7" = 1.5
  constraint coincident L0.start L3.end
  constraint perpendicular L0 L4
  constraint coincident L2.end L3.start
  constraint perpendicular L2 L5
  constraint perpendicular L5 L6
  constraint horizontal L7
  constraint vertical L8
  constraint horizontal L9
  constraint vertical L10
  measures "d5" distance of L0.start L4.end
  measures "d6" distance of L2.end L5.end
  measures "d7" distance of L5.end L6.end
extrude "Extrusion2" add sketch "Esquisse2" along normal blind 12
sketch "Esquisse3" plane through (0, 0, -1.5) normal (0, 0, -1) x (1, 0, 0)
  line L0 (-2, 0) -> (11.5, 0)
  line L1 (11.5, 0) -> (11.5, 12)
  line L2 (11.5, 12) -> (-2, 12)
  line L3 (-2, 12) -> (-2, 0)
  line L4 (-1.4002, 7.7) -> (-1.4002, 4.7)
  line L5 (-1.4002, 6.2) -> (11.0735, 6.2)
  line L6 (-1.0229, 4.2814) -> (0.6578, 4.2814)
  line L7 (4.728, 6.2) -> (4.728, 1.4574)
  line L8 (0.6578, 4.2814) -> (3.8134, 1.2287)
  arc A0 (-1.4002, 4.7) -> (-1.0229, 4.2814) centre (-0.9794, 4.7) ccw
  arc A1 (3.8134, 1.2287) -> (4.728, 1.4574) centre (4.2421, 1.4574) ccw
  arc A2 (5.414, 5.2875) -> (6.1572, 6.2) centre (5.2565, 6.1747) ccw
  arc A3 (5.414, 5.2875) -> (5.414, 4.3386) centre (5.6384, 4.8131) ccw
  arc A4 (5.414, 4.3386) -> (7.1239, 6.2) centre (5.3024, 6.1572) ccw
  arc A5 (6.4838, 3.698) -> (6.9788, 2.7993) centre (6.844, 3.3107) ccw
  arc A6 (6.4838, 3.698) -> (8.0468, 6.2) centre (5.3449, 6.1487) ccw
  arc A7 (6.9788, 2.7993) -> (9.0236, 6.2) centre (5.0787, 6.257) ccw
  arc A8 (7.5128, 2.3565) -> (7.9947, 1.4578) centre (7.8582, 1.9631) ccw
  arc A9 (7.5128, 2.3565) -> (9.9484, 6.2) centre (5.5404, 6.2998) ccw
  arc A10 (7.9947, 1.4578) -> (10.8862, 6.2) centre (5.6008, 6.17) ccw
  line L9 (-1.4002, 4.7) -> (-1.4002, 7.7)
  arc A11 (-1.0229, 8.1185) -> (-1.4002, 7.7) centre (-0.9794, 7.7) ccw
  line L10 (-1.0229, 8.1185) -> (0.6578, 8.1185)
  line L11 (0.6578, 8.1185) -> (3.8134, 11.1712)
  arc A12 (4.728, 10.9425) -> (3.8134, 11.1712) centre (4.2421, 10.9425) ccw
  line L12 (4.728, 6.2) -> (4.728, 10.9425)
  arc A13 (6.1572, 6.2) -> (5.414, 7.1124) centre (5.2565, 6.2252) ccw
  arc A14 (5.414, 8.0613) -> (5.414, 7.1124) centre (5.6384, 7.5868) ccw
  arc A15 (7.1239, 6.2) -> (5.414, 8.0613) centre (5.3024, 6.2427) ccw
  arc A16 (8.0468, 6.2) -> (6.4838, 8.7019) centre (5.3449, 6.2512) ccw
  arc A17 (6.9788, 9.6006) -> (6.4838, 8.7019) centre (6.844, 9.0892) ccw
  arc A18 (9.0236, 6.2) -> (6.9788, 9.6006) centre (5.0787, 6.1429) ccw
  arc A19 (9.9484, 6.2) -> (7.5128, 10.0434) centre (5.5404, 6.1001) ccw
  arc A20 (7.9947, 10.9421) -> (7.5128, 10.0434) centre (7.8582, 10.4368) ccw
  arc A21 (10.8862, 6.2) -> (7.9947, 10.9421) centre (5.6008, 6.2299) ccw
  dimension "d10" = 3
  constraint vertical L4
  constraint midpoint L4 L5.start
  constraint perpendicular L4 L5
  constraint horizontal L6
  constraint coincident L5 L7.start
  constraint perpendicular L5 L7
  constraint tangent L4 A0
  constraint tangent L7 A1
  constraint coincident L5 A2.end
  constraint coincident L5 A4.end
  constraint coincident L5 A6.end
  constraint coincident L5 A7.end
  constraint tangent A7 A9
  constraint coincident L5 A9.end
  constraint coincident L5 A10.end
  constraint symmetric L4.start L5 L4.end
  constraint symmetric L4.end L5 L4.start
  constraint symmetric L5 L6.start A11.start
  constraint symmetric L5 L6.end L10.end
  constraint symmetric L5 L7.start L12.start
  constraint symmetric L5 L7.end A12.start
  constraint symmetric L5 L8.end L11.end
  constraint symmetric L5 A0 A11
  constraint symmetric L5 A1 A12
  constraint symmetric L5 A2.end A13.start
  constraint symmetric L5 A2.start A13.end
  constraint symmetric L5 A2 A13
  constraint symmetric L5 A3.end A14.start
  constraint symmetric L5 A3 A14
  constraint symmetric L5 A4.end A15.start
  constraint symmetric L5 A4 A15
  constraint symmetric L5 A5.start A16.end
  constraint symmetric L5 A5.end A17.start
  constraint symmetric L5 A5 A17
  constraint symmetric L5 A6.end A16.start
  constraint symmetric L5 A6 A16
  constraint symmetric L5 A7.end A18.start
  constraint symmetric L5 A7 A18
  constraint symmetric L5 A8.start A19.end
  constraint symmetric L5 A8.end A20.start
  constraint symmetric L5 A8 A20
  constraint symmetric L5 A9.end A19.start
  constraint symmetric L5 A9 A19
  constraint symmetric L5 A10.end A21.start
  constraint symmetric L5 A10 A21
  measures "d10" distance of L4.start L4.end
extrude "Extrusion3" add sketch "Esquisse3" along normal blind 1 contours L4 L5 L9 A11 L10 L11 A12 L12 | L4 L5 L6 L7 L8 A0 A1 L9 | L5 A13 A14 A15 | L5 A2 A3 A4 | L5 A16 A17 A18 | L5 A5 A6 A7 | L5 A19 A20 A21 | L5 A8 A9 A10

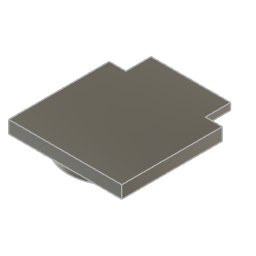
design "Etiquette_chrome"
Autodesk Fusion 360 part; units mm, degrees
sketch "Esquisse1" plane through (0, 0, 0) normal (0, 1, 0) x (1, 0, 0)
  line L0 (0, 0) -> (9.5, 0)
  line L1 (9.5, 0) -> (9.5, 0.8)
  line L2 (9.5, 0.8) -> (0, 0.8)
  line L3 (0, 0.8) -> (0, 0)
  dimension "d1" = 9.5
  dimension "d2" = 0.8
  constraint horizontal L0
  constraint vertical L1
  constraint horizontal L2
  constraint vertical L3
  constraint coincident L0.start L3.end
  measures "d1" distance of L0.start L0.end
  measures "d2" distance of L0.start L2.end
extrude "Extrusion1" add sketch "Esquisse1" along normal blind 3 makes body 1
sketch "Esquisse2" plane through (0, 0, 0) normal (0, -1, 0) x (1, 0, 0)
  line L0 (0, 0) -> (0, -0.8)
  line L1 (0, -0.8) -> (9.5, -0.8)
  line L2 (9.5, -0.8) -> (9.5, 0)
  line L3 (9.5, 0) -> (0, 0)
  line L4 (0, 0) -> (-2, 0) construction
  line L5 (9.5, 0) -> (11.5, 0)
  line L6 (11.5, 0) -> (11.5, -1.5)
  line L7 (-2, 0) -> (11.5, 0)
  line L8 (11.5, 0) -> (11.5, -1.5)
  line L9 (11.5, -1.5) -> (-2, -1.5)
  line L10 (-2, -1.5) -> (-2, 0)
  dimension "d5" = 2
  dimension "d6" = 2
  dimension "d7" = 1.5
  constraint coincident L0.start L3.end
  constraint perpendicular L0 L4
  constraint coincident L2.end L3.start
  constraint perpendicular L2 L5
  constraint perpendicular L5 L6
  constraint horizontal L7
  constraint vertical L8
  constraint horizontal L9
  constraint vertical L10
  measures "d5" distance of L0.start L4.end
  measures "d6" distance of L2.end L5.end
  measures "d7" distance of L5.end L6.end
extrude "Extrusion2" add sketch "Esquisse2" along normal blind 12 bodies 1